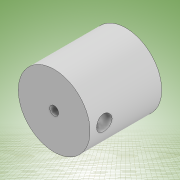
# Autodesk Inventor part: AcopleMotor
Saved by Autodesk Inventor 2022 (Build 260153000, 153)
## iProperties
Created: 2022-03-04
Part Number: AcopleMotor
Material: Genérico
Document SubType Name: Modeling
Designer: Marco
Density: 1 g/cm^3
Appearance: Valor por defecto
Author: Marco
Autodesk Inventor part; units mm, degrees
ref_plane "YZ Plane" through (0, 0, 0) normal (1, 0, 0) x (0, 1, 0)
ref_plane "XZ Plane" through (0, 0, 0) normal (0, 1, 0) x (-1, 0, 0)
ref_plane "XY Plane" through (0, 0, 0) normal (0, 0, 1) x (1, 0, 0)
sketch "Boceto1" plane through (0, 0, 0) normal (0, 0, 1) x (1, 0, 0)
  circle A0 centre (0, 0) radius 10
  dimension "d0" = 20
  constraints: 1 centre point, 1 coincident
  measures "d0" diameter of A0
extrude "Extrusión1" add sketch "Boceto1" along normal blind 20
sketch "Boceto2" plane through (0, 0, 20) normal (0, 0, 1) x (1, 0, 0)
  circle A0 centre (0, 0) radius 1.25
  dimension "d3" = 2.5
  constraints: 1 centre point, 1 coincident
  measures "d3" diameter of A0
extrude "Extrusión2" cut sketch "Boceto2" against normal blind 10
sketch "Boceto3" plane through (0, 0, 0) normal (0, 0, -1) x (-1, 0, 0)
  line L0 (0, 3.5218) -> (3.05, 1.7609)
  line L1 (3.05, 1.7609) -> (3.05, -1.7609)
  line L2 (3.05, -1.7609) -> (0, -3.5218)
  line L3 (0, -3.5218) -> (-3.05, -1.7609)
  line L4 (-3.05, -1.7609) -> (-3.05, 1.7609)
  line L5 (-3.05, 1.7609) -> (0, 3.5218)
  point P0 (0, 0)
  point P1 (0, 0)
  point P2 (3.05, 0)
  dimension "d6" = 6.1
  constraints: 12 end point, 1 coincident, 1 horizontal alignment, 1 midpoint, 13 other
  measures "d6" distance of L1.end L3.end
extrude "Extrusión3" cut sketch "Boceto3" against normal blind 10
ref_plane "Plano de trabajo1" through (10, 0, 0) normal (-1, 0, 0) x (0, 0, 1)
sketch "Boceto4" plane through (10, 0, 0) normal (-1, 0, 0) x (0, 0, 1)
  circle A0 centre (16, 0) radius 2
  line L0 (20, -10) -> (20, 10) projected
  point P0 (0, 0)
  dimension "d11" = 4
  dimension "d12" = 4
  constraints: 1 centre point, 1 horizontal alignment
  measures "d11" diameter of A0
  measures "d12" distance from line of L0 A0.centre
hole "Agujero1" at (10, 0, 16) direction (-1, 0, 0) diameter 4.3 end through all
